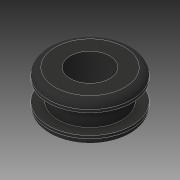
# Autodesk Inventor part: .5ID 1.0625OD Grommet (McMaster Carr #9307K63)
Saved by Autodesk Inventor 2021 (Build 250183000, 183)
## iProperties
Created: 2017-09-14
Part Number: .5ID 1.0625OD Grommet (McMaster Carr #9307K63)
Material: Rubber
Document SubType Name: Modeling
Density: 0.93 g/cm^3
Appearance: Rubber - Black
Mass: 3.68718 g
Surface Area: 26.515 cm^2
Volume: 3.96471 cm^3
Autodesk Inventor part; units mm, degrees
ref_plane "YZ Plane" through (0, 0, 0) normal (1, 0, 0) x (0, 1, 0)
ref_plane "XZ Plane" through (0, 0, 0) normal (0, 1, 0) x (-1, 0, 0)
ref_plane "XY Plane" through (0, 0, 0) normal (0, 0, 1) x (1, 0, 0)
sketch "Sketch1" plane through (0, 0, 0) normal (0, 0, 1) x (1, 0, 0)
  line L0 (0, 0) -> (0, 6.5039) construction
  line L1 (6.35, 6.35) -> (6.35, 0)
  line L2 (6.35, 0) -> (6.35, -6.35)
  line L3 (6.35, 6.35) -> (13.4937, 6.35)
  line L4 (13.4937, 6.35) -> (13.4937, 3.175)
  line L5 (13.4937, 3.175) -> (10.3188, 3.175)
  line L6 (10.3188, 3.175) -> (10.3188, -3.175)
  line L7 (10.3188, -3.175) -> (13.4937, -3.175)
  line L8 (13.4937, -3.175) -> (13.4937, -6.35)
  line L9 (13.4937, -6.35) -> (6.35, -6.35)
  dimension "d0" = 12.7
  dimension "d1" = 12.7
  dimension "d2" = 6.35
  dimension "d3" = 26.9875
  dimension "d4" = 20.6375
  constraints: 20 end point, 5 perpendicular, 4 equal length, 3 vertical, 1 horizontal, 1 horizontal alignment
  measures "d0" distance of L2.end L1.start
  measures "d1" diameter of L1 L0
  measures "d2" distance of L5.end L6.end
  measures "d3" diameter of L4 L0
  measures "d4" diameter of L6 L0
revolve "Revolution1" add sketch "Sketch1" angle 360 about axis through (0, 0, 0) along (0, 1, 0)
fillet "Fillet1" radius 2.286 2 edges at (-13.4937, 6.35, 0) (-13.4937, -6.35, 0)
body "Solid1"
